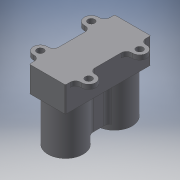
# Autodesk Inventor part: Side Lidar
Saved by Autodesk Inventor 2016 (Build 200138000, 138)
## iProperties
Created: 2017-05-14
Part Number: Side Lidar
Material: Generic
Document SubType Name: Modeling
Designer: BenjaPad
Density: 1 g/cm^3
Appearance: Default
Author: BenjaPad
Autodesk Inventor part; units mm, degrees
ref_plane "YZ Plane" through (0, 0, 0) normal (1, 0, 0) x (0, 1, 0)
ref_plane "XZ Plane" through (0, 0, 0) normal (0, 1, 0) x (-1, 0, 0)
ref_plane "XY Plane" through (0, 0, 0) normal (0, 0, 1) x (1, 0, 0)
sketch "Sketch1" plane through (0, 0, 0) normal (0, 0, 1) x (1, 0, 0)
  line L0 (10.25, 24.25) -> (10.25, -24.25) projected
  line L1 (-10.25, 24.25) -> (10.25, 24.25) projected
  line L2 (-10.25, -24.25) -> (-10.25, -9) projected
  line L3 (-10.25, 9) -> (-10.25, 24.25) projected
  line L4 (10.25, -24.25) -> (-10.25, -24.25) projected
  circle A0 centre (13.75, -14.5) radius 1.95 projected
  circle A1 centre (13.75, 14.5) radius 1.95 projected
  circle A2 centre (-13.75, 14.5) radius 1.95 projected
  circle A3 centre (-13.75, -14.5) radius 1.95 projected
  line L5 (-10.25, 9) -> (-10.25, -9)
  arc A4 (10.25, 12.5635) -> (10.25, 16.4365) centre (13.75, 14.5) ccw
  arc A5 (10.25, -16.4365) -> (10.25, -12.5635) centre (13.75, -14.5) ccw
  arc A6 (-10.25, -12.5635) -> (-10.25, -16.4365) centre (-13.75, -14.5) ccw
  arc A7 (-10.25, 16.4365) -> (-10.25, 12.5635) centre (-13.75, 14.5) ccw
  point P0 (0, 0)
  dimension "d0" = 8
  dimension "d1" = 8
  dimension "d2" = 8
  dimension "d3" = 8
  constraints: 8 point on circle, 8 point on line, 4 centre point, 4 coincident, 2 end point, 1 collinear
  measures "d0" diameter of A4
  measures "d1" diameter of A5
  measures "d2" diameter of A6
  measures "d3" diameter of A7
extrude "Extrusion1" add sketch "Sketch1" along normal blind 2.6
sketch "Sketch2" plane through (0, 0, 0) normal (0, 0, -1) x (-1, 0, 0)
  line L0 (10.25, 24.25) -> (10.25, 16.4365) projected
  line L1 (-10.25, -24.25) -> (-10.25, -16.4365) projected
  line L2 (10.25, 24.25) -> (-10.25, 24.25)
  line L3 (-10.25, 24.25) -> (-10.25, -24.25)
  line L4 (-10.25, -24.25) -> (10.25, -24.25)
  line L5 (10.25, -24.25) -> (10.25, 24.25)
  point P0 (0, 0)
  constraints: 8 end point, 2 parallel, 1 horizontal, 1 perpendicular
extrude "Extrusion2" add sketch "Sketch2" along normal blind 11.9
sketch "Sketch3" plane through (0, 0, -11.9) normal (0, 0, -1) x (-1, 0, 0)
  circle A0 centre (0, 13.9) radius 10 projected
  circle A1 centre (0, -13.9) radius 10 projected
  line L0 (4.85, 5.1549) -> (4.85, -5.1549)
  line L1 (-4.85, -5.1549) -> (-4.85, 5.1549)
  line L2 (-4.85, 7.8675) -> (4.85, -7.8675) construction
  line L3 (4.85, 7.8675) -> (-4.85, -7.8675) construction
  point P0 (0, 0)
  dimension "d8" = 9.7
  constraints: 8 end point, 4 point on circle, 2 midpoint, 1 parallel
  measures "d8" distance of L2.end L3.end
extrude "Extrusion3" add sketch "Sketch3" along normal blind 22
sketch "Sketch4" plane through (0, 0, -33.9) normal (0, 0, -1) x (-1, 0, 0)
  arc A0 (4.85, 5.1549) -> (-4.85, 5.1549) centre (0, 13.9) ccw projected
  circle A1 centre (0, 13.9) radius 10
  arc A2 (-4.85, -5.1549) -> (4.85, -5.1549) centre (0, -13.9) ccw projected
  circle A3 centre (0, -13.9) radius 10
  point P0 (0, 0)
  constraints: 2 centre point, 2 coincident
extrude "Extrusion4" add sketch "Sketch4" along normal blind 3
fillet "Fillet1" radius 4 4 edges at (-4.85, 5.1549, -22.9) (-4.85, -5.1549, -22.9) (4.85, -5.1549, -22.9) (4.85, 5.1549, -22.9)
fillet "Fillet2" radius 3 8 edges at (-10.25, -12.5635, 1.3) (-10.25, -16.4365, 1.3) (-10.25, 16.4365, 1.3) (-10.25, 12.5635, 1.3) (10.25, 12.5635, 1.3) (10.25, 16.4365, 1.3) (10.25, -16.4365, 1.3) (10.25, -12.5635, 1.3)
fillet "Fillet3" radius 0.5 4 edges at (-10.25, -24.25, -4.65) (10.25, -24.25, -4.65) (10.25, 24.25, -4.65) (-10.25, 24.25, -4.65)
body "Solid1"
